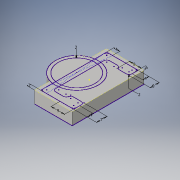
# Autodesk Inventor part: wide_access_platform_v01
Saved by Autodesk Inventor 2016 (Build 200138000, 138)
## iProperties
Company: HMS
Created: 2016-07-11
Part Number: wide_access_platform_v01
Material: Generic
Document SubType Name: Modeling
Designer: Stephen Holtz
Density: 1 g/cm^3
Appearance: Default
Author: Stephen Holtz
Title: Wide Access Drosophila Physiology Platform
Autodesk Inventor part; units mm, degrees
ref_plane "YZ Plane" through (0, 0, 0) normal (1, 0, 0) x (0, 1, 0)
ref_plane "XZ Plane" through (0, 0, 0) normal (0, 1, 0) x (-1, 0, 0)
ref_plane "XY Plane" through (0, 0, 0) normal (0, 0, 1) x (1, 0, 0)
sketch "Sketch2" plane through (0, 0, 0) normal (0, 1, 0) x (-1, 0, 0)
  line L0 (12.5, 24) -> (12.5, -24)
  line L1 (12.5, -24) -> (-12.5, -24)
  line L2 (-12.5, -24) -> (-12.5, 24)
  line L3 (-12.5, 24) -> (12.5, 24)
  line L4 (12.5, 24) -> (-12.5, -24) construction
  line L5 (12.5, -24) -> (-12.5, 24) construction
  line L6 (8.5, 24) -> (8.5, -24)
  circle A0 centre (8.5, 0) radius 14.25
  point P0 (0, 0)
  dimension "d9" = 25
  dimension "d10" = 48
  dimension "d11" = 4
  dimension "d12" = 28.5
  constraints: 14 end point, 3 midpoint, 2 parallel, 2 perpendicular, 2 point on line, 1 centre point, 1 vertical
  measures "d9" distance of L0.end L1.end
  measures "d10" distance of L1.end L2.end
  measures "d11" distance between parallel lines of L0 L6
  measures "d12" diameter of A0
extrude "Extrusion2" add sketch "Sketch2" along normal blind 8
sketch "Sketch3" plane through (0, 8, 0) normal (0, 1, 0) x (1, 0, 0)
  arc A0 (-12.5, 13.6771) -> (-12.5, -13.6771) centre (-8.5, 0) ccw construction
  line L0 (-12.5, -13.6771) -> (-12.5, -24) construction
  line L1 (-12.5, -24) -> (12.5, -24) construction
  line L2 (12.5, -24) -> (12.5, 24) construction
  line L3 (12.5, 24) -> (-12.5, 24) construction
  line L4 (-12.5, 24) -> (-12.5, 13.6771) construction
  circle A1 centre (-8.5, 0) radius 14.25 construction
  circle A2 centre (-8.5, 0) radius 14.25
  circle A3 centre (-8.5, 0) radius 12.25
  line L5 (-6.5, -22) -> (-8.5, -22)
  line L6 (-10.5, -22) -> (-10.5, 22)
  line L7 (-10.5, 22) -> (-6.5, 22)
  line L8 (-6.5, 16) -> (-6.5, -16)
  line L9 (-6.5, -22) -> (-10.5, 22) construction
  line L10 (-10.5, -22) -> (-6.5, 22) construction
  line L11 (-8.5, 22) -> (10.5, 22)
  line L12 (10.5, 20) -> (10.5, 18)
  line L13 (0.5, 18) -> (-4.5, 18)
  line L14 (-10.5, 18) -> (-10.5, 20)
  line L15 (-10.5, -22) -> (9.5, -22)
  line L16 (11.5, -20) -> (11.5, -18)
  line L17 (0.5, -18) -> (-4.5, -18)
  line L18 (-10.5, -18) -> (-10.5, -20)
  line L19 (8.5, 22) -> (2.5, 22)
  line L20 (2.5, 16) -> (2.5, 16)
  line L21 (3.9641, 16) -> (8.5, 16)
  line L22 (10.5, 18) -> (10.5, 22)
  line L23 (11.5, -22) -> (2.5, -22)
  line L24 (2.5, -16) -> (2.5, -17)
  line L25 (4.5, -15) -> (9.5, -15)
  line L26 (11.5, -17) -> (11.5, -22)
  arc A4 (8.5, 16) -> (10.5, 18) centre (8.5, 18) ccw
  arc A5 (10.5, 20) -> (8.5, 22) centre (8.5, 20) ccw
  arc A6 (-8.5, 22) -> (-10.5, 20) centre (-8.5, 20) ccw
  arc A7 (-10.5, -20) -> (-8.5, -22) centre (-8.5, -20) ccw
  arc A8 (9.5, -22) -> (11.5, -20) centre (9.5, -20) ccw
  arc A9 (11.5, -17) -> (9.5, -15) centre (9.5, -17) ccw
  arc A10 (4.5, -15) -> (2.5, -17) centre (4.5, -17) ccw
  arc A11 (-6.5, -16) -> (-4.5, -18) centre (-4.5, -16) ccw
  arc A12 (0.5, -18) -> (2.5, -16) centre (0.5, -16) ccw
  arc A13 (2.2321, 17) -> (0.5, 18) centre (0.5, 16) ccw
  arc A14 (-4.5, 18) -> (-6.5, 16) centre (-4.5, 16) ccw
  arc A15 (2.2321, 17) -> (3.9641, 16) centre (3.9641, 18) ccw
  point P0 (0, 0)
  point P1 (10.5, 16)
  point P2 (2.5, -15)
  point P3 (11.5, -15)
  dimension "recess_dist" = 2
  dimension "d16" = 4
  dimension "d17" = 2
  dimension "d18" = 4
  dimension "d19" = 4
  dimension "d20" = 6
  dimension "d21" = 7
  dimension "d22" = 9
  dimension "d23" = 2
  dimension "d24" = 8
  dimension "d25" = 2
  constraints: 44 end point, 25 point on circle, 24 point on line, 24 tangent, 14 centre point, 12 equal radius, 10 parallel, 5 horizontal, 5 perpendicular, 2 coincident, 2 midpoint
  measures "recess_dist" radial gap between concentric circles of A1 A3
  measures "d16" distance of L6.end L7.end
  measures "d17" distance between parallel lines of L1 L5
  measures "d18" distance of L11.end L12.end
  measures "d19" distance of L23.start L16.end
  measures "d20" distance of point (10.5, 16) L11.end
  measures "d21" distance of point (11.5, -15) L23.start
  measures "d22" distance of L23.start L23.end
  measures "d23" distance between parallel lines of L2 L22
  measures "d24" distance between parallel lines of L12 L20
  measures "d25" radius of A4
body "Solid2"
